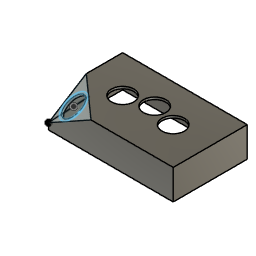
test_mount (Autodesk Fusion 360 design; units mm, degrees)
Autodesk Fusion 360 part; units mm, degrees
note: some values were not read from the file. Set by a fixed rule: which face or edge a step refers to.
sketch "Sketch1" plane through (0, 0, 0) normal (0, 0, 1) x (1, 0, 0)
  circle A0 centre (0, 0) radius 15
  line L0 (0, 0) -> (33.8074, 9.0587)
  line L1 (0, 0) -> (35, 0) construction
  line L2 (33.8074, 9.0587) -> (67.6148, 0)
  line L3 (33.8074, 9.0587) -> (69.4683, 9.0587) construction
  circle A1 centre (33.8074, 9.0587) radius 15
  circle A2 centre (67.6148, 0) radius 15
  circle A3 centre (0, 0) radius 17.5
  circle A4 centre (33.8074, 9.0587) radius 17.5
  circle A5 centre (67.6148, 0) radius 17.5
  line L4 (0, 0) -> (-49.4975, -49.4975)
  line L5 (0, 0) -> (50, 0) construction
  line L6 (67.6148, 0) -> (117.1123, 49.4975)
  line L7 (67.6148, 0) -> (117.6148, 0) construction
  line L8 (-49.4975, -49.4975) -> (117.1123, -49.4975)
  line L9 (117.1123, -49.4975) -> (117.1123, 49.4975)
  line L10 (117.1123, 49.4975) -> (-49.4975, 49.4975)
  line L11 (-49.4975, 49.4975) -> (-49.4975, -49.4975)
  dimension "d1" = 30
  dimension "d2" = 35
  dimension "d3" = 15
  dimension "d4" = 15
  dimension "d5" = 35
  dimension "d6" = 30
  dimension "d7" = 30
  dimension "d8" = 35
  dimension "d9" = 35
  dimension "d10" = 35
  dimension "d11" = 135
  dimension "d12" = 70
  dimension "d13" = 45
  dimension "d14" = 70
  constraint coincident A0.centre L0.start
  constraint horizontal L1
  constraint horizontal L3
  constraint coincident L0.end L2.start
  constraint coincident L2.end A2.centre
  constraint concentric A0 A3
  constraint concentric A1 A4
  constraint concentric A2 A5
  constraint horizontal L5
  constraint horizontal L7
  constraint horizontal L8
  constraint vertical L9
  constraint horizontal L10
  constraint vertical L11
  measures "d1" diameter of A0
  measures "d2" distance of A0.centre L0.end
  measures "d3" angle of L0 L1
  measures "d4" angle of L2 L3
  measures "d5" distance of L0.end L2.end
  measures "d6" diameter of A1
  measures "d7" diameter of A2
  measures "d8" diameter of A3
  measures "d9" diameter of A4
  measures "d10" diameter of A5
  measures "d11" angle of L4 L5
  measures "d12" distance of A0.centre L4.end
  measures "d13" angle of L6 L7
  measures "d14" distance of L2.end L6.end
extrude "Extrude1" add sketch "Sketch1" against normal blind 40
sketch "Sketch2" plane through (0, 0, -40) normal (0, 0, -1) x (1, 0, 0)
  line L0 (-49.4975, 49.4975) -> (-49.4975, -49.4975)
  line L1 (-49.4975, -49.4975) -> (117.1123, -49.4975)
  line L2 (117.1123, -49.4975) -> (117.1123, 49.4975)
  line L3 (117.1123, 49.4975) -> (-49.4975, 49.4975)
  line L4 (-49.4975, 49.4975) -> (117.1123, 49.4975)
  line L5 (117.1123, 49.4975) -> (117.1123, -49.4975)
  line L6 (117.1123, -49.4975) -> (-49.4975, -49.4975)
  line L7 (-49.4975, -49.4975) -> (-49.4975, 49.4975)
  line L8 (-49.4975, 49.4975) -> (-46.4975, 49.4975)
  line L9 (-46.4975, 49.4975) -> (-46.4975, 46.4975)
  line L10 (-46.4975, 46.4975) -> (-49.4975, 46.4975)
  line L11 (-49.4975, 46.4975) -> (-49.4975, 49.4975)
  line L12 (117.1123, -49.4975) -> (114.1123, -49.4975)
  line L13 (114.1123, -49.4975) -> (114.1123, -46.4975)
  line L14 (114.1123, -46.4975) -> (117.1123, -46.4975)
  line L15 (117.1123, -46.4975) -> (117.1123, -49.4975)
  line L16 (-46.4975, 46.4975) -> (114.1123, 46.4975)
  line L17 (114.1123, 46.4975) -> (114.1123, -46.4975)
  line L18 (114.1123, -46.4975) -> (-46.4975, -46.4975)
  line L19 (-46.4975, -46.4975) -> (-46.4975, 46.4975)
  dimension "d17" = 3
  dimension "d18" = 3
  dimension "d19" = 3
  dimension "d20" = 3
  constraint horizontal L4
  constraint vertical L5
  constraint horizontal L6
  constraint vertical L7
  constraint coincident L1.end L2.start
  constraint coincident L0.start L3.end
  constraint horizontal L8
  constraint vertical L9
  constraint horizontal L10
  constraint vertical L11
  constraint horizontal L12
  constraint vertical L13
  constraint horizontal L14
  constraint vertical L15
  constraint horizontal L16
  constraint vertical L17
  constraint horizontal L18
  constraint vertical L19
  measures "d17" distance of L0.start L8.end
  measures "d18" distance of L0.start L10.end
  measures "d19" distance of L1.end L12.end
  measures "d20" distance of L1.end L14.end
sketch "Sketch3" plane through (0, -49.4975, 0) normal (0, -1, 0) x (1, 0, 0)
  line L0 (117.1123, 0) -> (-49.4975, 0)
  line L1 (-49.4975, 0) -> (-49.4975, -40)
  line L2 (-49.4975, -40) -> (117.1123, -40)
  line L3 (117.1123, -40) -> (117.1123, 0)
  line L4 (-49.4975, 0) -> (-14.4975, 0)
  line L5 (-14.4975, 0) -> (-14.4975, -25)
  line L6 (-14.4975, -25) -> (-49.4975, -25)
  line L7 (-49.4975, -25) -> (-49.4975, 0)
  dimension "d21" = 35
  dimension "d22" = 25
  constraint horizontal L4
  constraint vertical L5
  constraint horizontal L6
  constraint vertical L7
  constraint coincident L0.end L1.start
  measures "d21" distance of L0.end L4.end
  measures "d22" distance of L0.end L6.end
sketch "Sketch4" plane through (0, 0, 0) normal (0, 0, 1) x (-1, 0, 0)
  line L0 (49.4975, -49.4975) -> (49.4975, 49.4975)
  line L1 (49.4975, 49.4975) -> (-117.1123, 49.4975)
  line L2 (-117.1123, 49.4975) -> (-117.1123, -49.4975)
  line L3 (-117.1123, -49.4975) -> (49.4975, -49.4975)
  line L4 (49.4975, 49.4975) -> (4.4975, 49.4975)
  line L5 (4.4975, 49.4975) -> (4.4975, 9.4975)
  line L6 (4.4975, 9.4975) -> (49.4975, 9.4975)
  line L7 (49.4975, 9.4975) -> (49.4975, 49.4975)
  dimension "d23" = 45
  dimension "d24" = 40
  constraint horizontal L4
  constraint vertical L5
  constraint horizontal L6
  constraint vertical L7
  constraint coincident L0.end L1.start
  measures "d23" distance of L0.end L4.end
  measures "d24" distance of L0.end L6.end
sketch "Sketch5" plane through (-49.4975, 0, 0) normal (-1, 0, 0) x (0, -1, 0)
  line L0 (49.4975, 0) -> (-49.4975, 0)
  line L1 (-49.4975, 0) -> (-49.4975, -40)
  line L2 (-49.4975, -40) -> (49.4975, -40)
  line L3 (49.4975, -40) -> (49.4975, 0)
  line L4 (49.4975, 0) -> (4.4975, 0)
  line L5 (4.4975, 0) -> (4.4975, -25)
  line L6 (4.4975, -25) -> (49.4975, -25)
  line L7 (49.4975, -25) -> (49.4975, 0)
  dimension "d25" = 45
  dimension "d26" = 25
  constraint horizontal L4
  constraint vertical L5
  constraint horizontal L6
  constraint vertical L7
  constraint coincident L0.start L3.end
  measures "d25" distance of L0.start L4.end
  measures "d26" distance of L0.start L6.end
ref_plane "WorkPlane1" through (-4.4975, -49.4975, 0) normal (-0.426184, -0.479456, 0.76713) x (0.747409, -0.664364, 0)
sketch "Sketch7" plane through (-10.931, -12.2974, 19.6758) normal (-0.426184, -0.479456, 0.76713) x (0.725063, -0.688142, -0.027276)
  line L0 (-78.171, 22.0517) -> (87.1049, 22.0517)
  line L1 (87.1049, 22.0517) -> (87.1049, -109.6946)
  line L2 (87.1049, -109.6946) -> (-78.171, -109.6946)
  line L3 (-78.171, -109.6946) -> (-78.171, 22.0517)
  constraint horizontal L0
  constraint vertical L1
  constraint horizontal L2
  constraint vertical L3
extrude "Extrude2" cut sketch "Sketch7" along normal blind 70
extrude "Extrude3" cut sketch "Sketch7" against normal blind 5
sketch "Sketch10" plane through (-8.8001, -9.9001, 15.8402) normal (-0.426184, -0.479456, 0.76713) x (0.747409, -0.664364, 0)
  line L0 (38.2915, -24.6928) -> (-37.6134, -24.6928)
  line L1 (-37.6134, -24.6928) -> (-4.1105, -73.8249)
  line L2 (-4.1105, -73.8249) -> (38.2915, -24.6928)
  line L3 (-4.1105, -73.8249) -> (0.3391, -24.6928)
  circle A0 centre (-1.3238, -43.0538) radius 17.5
  circle A1 centre (-1.3238, -43.0538) radius 15
  dimension "d35" = 35
  dimension "d36" = 30
  constraint coincident L1.end L2.start
  constraint midpoint L0 L3.end
  constraint coincident L3 A0.centre
  constraint concentric A0 A1
  measures "d35" diameter of A0
  measures "d36" diameter of A1
shell "Shell1" thickness 3 removed faces 1 at (6.0391, 16.4992, -40)
extrude "Extrude6" cut sketch "Sketch1" against normal up to surface (3 mm away) contours A0 L0 L4 | A0 L0 L4 | L0 L2 A1 | L0 L2 A1 | L2 A2 L6 | L2 A2 L6
extrude "Extrude7" cut sketch "Sketch10" against normal up to surface (3 mm away) contours L3 A1 | L3 A1
